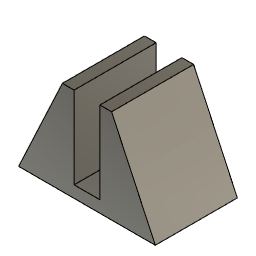
MotorHolder v4 (Autodesk Fusion 360 design; units mm, degrees)
Autodesk Fusion 360 part; units mm, degrees
box "BoxPrimitive1" add length 35 width 35 height 5 placed x (0, 1, 0) y (-1, 0, 0) z (0, 0, 1) at (35, 0, 0) makes body 1
copy_body "CopyPasteBodies1" bodies 1 makes body 2
move_body "Move1" bodies 2 to x (0, 0, 1) y (0, 1, 0) z (-1, 0, 0) at (0, 0, 0)
copy_body "CopyPasteBodies2" bodies 2 makes body 3
move_body "Move2" bodies 3 to x (0, 0, 1) y (0, 1, 0) z (-1, 0, 0) at (-5, 0, 5)
move_body "Move3" bodies 3 to x (1, 0, 0) y (0, 1, 0) z (0, 0, 1) at (0, 0, 11)
move_body "Move4" bodies 3 to x (1, 0, 0) y (0, 1, 0) z (0, 0, 1) at (40, 0, 0)
move_body "Move5" bodies 3 to x (1, 0, 0) y (0, 1, 0) z (0, 0, 1) at (0, 0, 6)
move_body "Move6" bodies 3 to x (1, 0, 0) y (0, 1, 0) z (0, 0, 1) at (0, 0, -1)
extrude "Extrude1" cut 1 faces at (-1.6667, 23.3333, 35) along direction (0, 0, -1) blind 14 on bodies 2 bodies 2
combine "Combine1" operation add target body 3 tool bodies 2 1
move_body "Move7" bodies 3 to x (1, 0, 0) y (0, 1, 0) z (0, 0, 1) at (0, 0, 20)
draft "Draft1" angle 25 neutral plane through (35, 0, 20) pull (1, 0, 0) 1 faces at (21.6667, 23.3333, 20) on bodies 3
move_body "Move8" bodies 3 to x (0, 0, 1) y (0, 1, 0) z (-1, 0, 0) at (-3.6523, 0, 6.3477)
draft "Draft2" angle 25 neutral plane through (-44.6523, 0, 41.3477) pull (0, 0, 1) 1 faces at (-44.6523, 11.6667, 28.0144) on bodies 3
